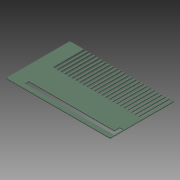
# Autodesk Inventor part: subrack_frontpanel
Saved by Autodesk Inventor 2015 (Build 190159000, 159)
## iProperties
Created: 2014-08-23
Part Number: subrack_frontpanel
Material: Aluminum
Document SubType Name: Modeling
Designer: Patrick Camilleri
Density: 2.7 g/cm^3
Appearance: Rubber - Green
Author: Patrick Camilleri
Autodesk Inventor part; units mm, degrees
ref_plane "YZ Plane" through (0, 0, 0) normal (1, 0, 0) x (0, 1, 0)
ref_plane "XZ Plane" through (0, 0, 0) normal (0, 1, 0) x (-1, 0, 0)
ref_plane "XY Plane" through (0, 0, 0) normal (0, 0, 1) x (1, 0, 0)
sketch "Sketch1" plane through (0, 0, 0) normal (0, 0, 1) x (1, 0, 0)
  line L0 (0, 0) -> (426.6, 0)
  line L1 (426.6, 0) -> (426.6, 261.454)
  line L2 (426.6, 261.454) -> (0, 261.454)
  line L3 (0, 261.454) -> (0, 0)
  point P0 (2.48, 2.8)
  point P1 (2.48, 258.65)
  dimension "d0" = 426.6
  dimension "d1" = 261.454
  dimension "d2" = 2.8
  dimension "d3" = 2.48
  dimension "d4" = 255.85
  dimension "d5" = 2.48
  constraints: 8 end point, 2 parallel, 1 horizontal, 1 perpendicular
  measures "d0" distance of L2.end L1.end
  measures "d1" distance of L1.end L0.end
  measures "d2" distance from line of L0 point (2.48, 2.8)
  measures "d3" distance from line of L3 point (2.48, 2.8)
  measures "d4" distance of point (2.48, 258.65) point (2.48, 2.8)
  measures "d5" distance from line of point (2.48, 258.65) L3
extrude "Extrusion1" add sketch "Sketch1" along normal blind 3
sketch "Sketch3" plane through (0, 0, 3) normal (0, 0, 1) x (1, 0, 0)
  line L0 (0, 261.454) -> (0, 0) projected
  line L1 (426.6, 0) -> (426.6, 261.454) projected
  line L2 (0, 0) -> (426.6, 0) projected
  line L3 (426.6, 261.454) -> (0, 261.454) projected
  line L4 (423.3, 19.2) -> (58.5, 19.2)
  line L5 (58.5, 19.2) -> (58.5, 35.2)
  line L6 (58.5, 35.2) -> (423.3, 35.2)
  line L7 (423.3, 35.2) -> (423.3, 19.2)
  line L8 (423.3, 35.2) -> (408.8, 35.2)
  line L9 (408.8, 35.2) -> (408.8, 57.7)
  line L10 (408.8, 57.7) -> (423.3, 57.7)
  line L11 (423.3, 57.7) -> (423.3, 35.2)
  dimension "d22" = 364.8
  dimension "d23" = 16
  dimension "d24" = 19.2
  dimension "d25" = 3.3
  dimension "d26" = 14.5
  dimension "d30" = 38.5
  constraints: 16 end point, 4 parallel, 2 collinear, 2 horizontal, 2 perpendicular
  measures "d22" distance of L5.end L6.end
  measures "d23" distance of L4.end L5.end
  measures "d24" distance between parallel lines of L2 L4
  measures "d25" distance between parallel lines of L1 L7
  measures "d26" distance of L10.end L9.end
  measures "d30" distance between parallel lines of L10 L4
extrude "Extrusion2" cut sketch "Sketch3" against normal blind 3 contours L4 L5 L6 L7 | L6 L9 L10 L11
sketch "Sketch4" plane through (0, 0, 3) normal (0, 0, 1) x (1, 0, 0)
  line L0 (426.6, 261.454) -> (0, 261.454) projected
  line L1 (426.6, 0) -> (426.6, 261.454) projected
  line L2 (0, 0) -> (426.6, 0) projected
  line L3 (408.8, 35.2) -> (408.8, 57.7) projected
  line L4 (408.8, 134) -> (417.3, 134)
  line L5 (417.3, 134) -> (417.3, 261.454)
  line L6 (417.3, 261.454) -> (408.8, 261.454)
  line L7 (408.8, 261.454) -> (408.8, 134)
  dimension "d36" = 8.5
  dimension "d38" = 134
  constraints: 8 end point, 2 collinear, 2 parallel, 1 horizontal, 1 perpendicular
  measures "d36" distance of L5.end L6.end
  measures "d38" distance between parallel lines of L4 L2
extrude "Extrusion3" cut sketch "Sketch4" against normal blind 3
pattern_linear "Rectangular Pattern2" count 24 spacing 15.24 along (-1, 0, 0) of "Extrusion3"
sketch "Sketch2" plane through (0, 0, 3) normal (0, 0, 1) x (1, 0, 0)
  line L0 (0, 261.454) -> (0, 0) projected
  line L1 (0, 0) -> (426.6, 0) projected
  line L2 (426.6, 261.454) -> (0, 261.454) projected
  line L3 (426.6, 0) -> (426.6, 261.454) projected
  point P0 (2.48, 2.8)
  point P1 (3.48, 258.648)
  point P2 (109.16, 2.8)
  point P3 (215.84, 2.8)
  point P4 (322.52, 2.8)
  point P5 (424.12, 2.8)
  point P6 (54.28, 258.648)
  point P7 (145.72, 258.648)
  point P8 (237.16, 258.648)
  point P9 (328.6, 258.648)
  point P10 (420.04, 258.648)
  dimension "d8" = 2.48
  dimension "d9" = 2.8
  dimension "d10" = 255.85
  dimension "d11" = 3.48
  dimension "d57" = 106.68
  dimension "d62" = 421.64
  dimension "d63" = 50.8
  dimension "d66" = 91.44
  constraints: 2 horizontal, 2 horizontal alignment, 7 other
  measures "d8" distance from line of L0 point (2.48, 2.8)
  measures "d9" distance from line of L1 point (2.48, 2.8)
  measures "d10" distance of point (3.48, 258.648) point (2.48, 2.8)
  measures "d11" distance from line of L0 point (3.48, 258.648)
  measures "d57" distance of point (2.48, 2.8) point (109.16, 2.8)
  measures "d62" distance of point (424.12, 2.8) point (2.48, 2.8)
  measures "d63" distance of point (54.28, 258.648) point (3.48, 258.648)
  measures "d66" distance of point (54.28, 258.648) point (145.72, 258.648)
hole "Hole1" at (2.48, 2.8, 3) at (3.48, 258.648, 3) at (109.16, 2.8, 3) at (215.84, 2.8, 3) at (322.52, 2.8, 3) at (424.12, 2.8, 3) at (420.04, 258.648, 3) at (145.72, 258.648, 3) at (237.16, 258.648, 3) at (328.6, 258.648, 3) at (54.28, 258.648, 3) direction (0, 0, -1) diameter 2.5 end through all
equation "\"d5\" = d3"
body "Solid1"
